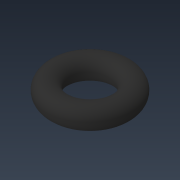
# Autodesk Inventor part: O-Ring 6x4.0
Saved by Autodesk Inventor 2022.1 (Build 261234020, 234B)
## iProperties
Part Number: O-Ring 6x4.0
Material: Gummi, Silikon
Document SubType Name: Modeling
Designer: rYan
Density: 1.25 g/cm^3
Appearance: Gummi - schwarz
Mass: 0.542828 g
Surface Area: 4.34263 cm^2
Volume: 0.434263 cm^3
Author: rYan
Autodesk Inventor part; units mm, degrees
ref_plane "YZ Plane" through (0, 0, 0) normal (1, 0, 0) x (0, 1, 0)
ref_plane "XZ Plane" through (0, 0, 0) normal (0, 1, 0) x (-1, 0, 0)
ref_plane "XY Plane" through (0, 0, 0) normal (0, 0, 1) x (1, 0, 0)
sketch "Skizze1" plane through (0, 0, 0) normal (1, 0, 0) x (0, 1, 0)
  line L0 (0, 1.1382) -> (0, -1.1246)
  circle A0 centre (-5.5, 0) radius 2
  line L1 (-9, 0) -> (1.5, 0) projected
  line L2 (-3.5, 0.8713) -> (-3.5, -0.7181) construction
  point P0 (0, 0)
  dimension "d0" = 4
  dimension "d3" = 7
  constraints: 4 end point, 2 point on line, 2 vertical, 1 centre point, 1 tangent
  measures "d0" diameter of A0
  measures "d3" diameter of L2 L0
revolve "Umdrehung1" add sketch "Skizze1" angle 360 about axis through (0, 0, 1.1382) along (0, 0, -1)
